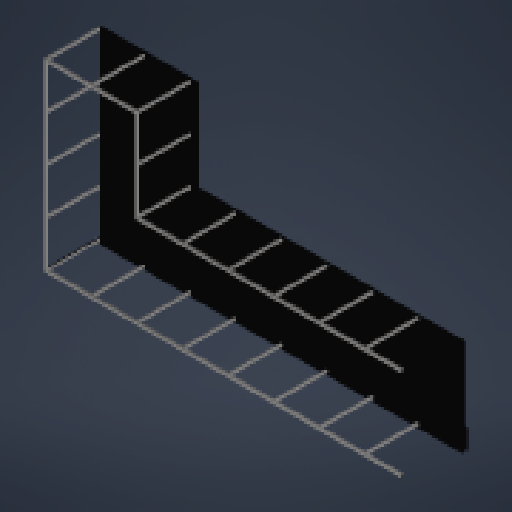
# Autodesk Inventor part: FirstFloorP
Saved by Autodesk Inventor 2025 (Build 290162000, 162)
## iProperties
Created: 2024-05-05
Part Number: FirstFloorP
Material: Generic
Document SubType Name: Modeling
Designer: zulet
Density: 1 g/cm^3
Appearance: Black
Author: zulet
Autodesk Inventor part; units mm, degrees
ref_plane "YZ Plane" through (0, 0, 0) normal (1, 0, 0) x (0, 1, 0)
ref_plane "XZ Plane" through (0, 0, 0) normal (0, 1, 0) x (-1, 0, 0)
ref_plane "XY Plane" through (0, 0, 0) normal (0, 0, 1) x (1, 0, 0)
sketch "Sketch1" plane through (0, 0, 0) normal (0, 0, 1) x (1, 0, 0)
  line L0 (7383.4617, 1848.5139) -> (5993.4617, 1848.5139) projected
  line L1 (7383.4617, 3293.5139) -> (7383.4617, 1793.5139) projected
  line L2 (7383.4617, 653.5139) -> (7383.4617, 1793.5139) projected
  line L3 (7353.4617, 653.5139) -> (7523.4617, 653.5139) projected
  line L4 (7416.4617, 640.8139) -> (7353.4617, 640.8139) projected
  arc A0 (7434.4617, 622.8139) -> (7416.4617, 640.8139) centre (7416.4617, 622.8139) ccw projected
  line L5 (7353.4617, 640.8139) -> (7353.4617, 653.5139) projected
  line L6 (7434.4617, 324.2139) -> (7434.4617, 622.8139) projected
  arc A1 (7416.4617, 306.2139) -> (7434.4617, 324.2139) centre (7416.4617, 324.2139) ccw projected
  line L7 (7416.4617, 306.2139) -> (7353.4617, 306.2139) projected
  line L8 (5938.4617, 348.5139) -> (7353.4617, 348.5139) construction
  line L9 (7353.4617, 238.5139) -> (7353.4617, 348.5139) projected
  line L10 (5938.4617, 238.5139) -> (7353.4617, 238.5139) projected
  line L11 (4438.4617, 238.5139) -> (5938.4617, 238.5139) projected
  line L12 (4438.4617, 238.5139) -> (2938.4617, 238.5139) projected
  line L13 (1438.4617, 238.5139) -> (2938.4617, 238.5139) projected
  line L14 (1383.4617, 1738.5139) -> (1383.4617, 348.5139) projected
  line L15 (1438.4617, 238.5139) -> (1438.4617, 348.5139) projected
  line L16 (1383.4617, 348.5139) -> (1493.4617, 348.5139) projected
  line L17 (1383.4617, 3238.5139) -> (1383.4617, 1848.5139) projected
  line L18 (2993.4617, 3348.5139) -> (1493.4617, 3348.5139) projected
  line L19 (2993.4617, 3238.5139) -> (2993.4617, 1848.5139) projected
  line L20 (2993.4617, 1848.5139) -> (4383.4617, 1848.5139) projected
  line L21 (4493.4617, 1848.5139) -> (5883.4617, 1848.5139) projected
  line L22 (1493.4617, 3348.5139) -> (1383.4617, 3348.5139)
  line L23 (1383.4617, 3348.5139) -> (1383.4617, 3238.5139)
  line L24 (1383.4617, 348.5139) -> (1383.4617, 238.5139)
  line L25 (1383.4617, 238.5139) -> (1438.4617, 238.5139)
  line L26 (2993.4617, 3348.5139) -> (2993.4617, 3238.5139)
  line L27 (4383.4617, 1848.5139) -> (4493.4617, 1848.5139)
  line L28 (5883.4617, 1848.5139) -> (5993.4617, 1848.5139)
  line L29 (1383.4617, 1848.5139) -> (1383.4617, 1738.5139)
  point P0 (0, 0)
  point P1 (7383.042, 1848.5139)
  point P2 (1472.0731, 342.554)
  constraints: 16 end point, 4 perpendicular, 1 collinear, 1 horizontal, 1 point on line, 1 vertical
extrude "Extrusion1" add sketch "Sketch1" along normal blind 20
sketch "Sketch2" plane through (0, 0, 20) normal (0, 0, 1) x (1, 0, 0)
  arc A0 (1423.4617, 286.5139) -> (1431.4617, 278.5139) centre (1431.4617, 286.5139) ccw projected
  line L0 (1423.4617, 286.5139) -> (1423.4617, 310.5139) projected
  arc A1 (1431.4617, 318.5139) -> (1423.4617, 310.5139) centre (1431.4617, 310.5139) ccw projected
  line L1 (1431.4617, 318.5139) -> (1455.4617, 318.5139) projected
  arc A2 (1463.4617, 310.5139) -> (1455.4617, 318.5139) centre (1455.4617, 310.5139) ccw projected
  line L2 (1463.4617, 310.5139) -> (1463.4617, 286.5139) projected
  arc A3 (1455.4617, 278.5139) -> (1463.4617, 286.5139) centre (1455.4617, 286.5139) ccw projected
  line L3 (1455.4617, 278.5139) -> (1431.4617, 278.5139) projected
  line L4 (1431.4617, 318.5139) -> (1455.4617, 318.5139)
  line L5 (1463.4617, 310.5139) -> (1463.4617, 286.5139)
  line L6 (1455.4617, 278.5139) -> (1431.4617, 278.5139)
  line L7 (1423.4617, 286.5139) -> (1423.4617, 310.5139)
  arc A4 (1431.4617, 318.5139) -> (1423.4617, 310.5139) centre (1431.4617, 310.5139) ccw
  arc A5 (1463.4617, 310.5139) -> (1455.4617, 318.5139) centre (1455.4617, 310.5139) ccw
  arc A6 (1455.4617, 278.5139) -> (1463.4617, 286.5139) centre (1455.4617, 286.5139) ccw
  arc A7 (1423.4617, 286.5139) -> (1431.4617, 278.5139) centre (1431.4617, 286.5139) ccw
  arc A8 (2205.4617, 278.5139) -> (2213.4617, 286.5139) centre (2205.4617, 286.5139) ccw
  line L8 (2205.4617, 278.5139) -> (2181.4617, 278.5139)
  line L9 (2213.4617, 310.5139) -> (2213.4617, 286.5139)
  arc A9 (2213.4617, 310.5139) -> (2205.4617, 318.5139) centre (2205.4617, 310.5139) ccw
  line L10 (2173.4617, 286.5139) -> (2173.4617, 310.5139)
  line L11 (2181.4617, 318.5139) -> (2205.4617, 318.5139)
  arc A10 (2181.4617, 318.5139) -> (2173.4617, 310.5139) centre (2181.4617, 310.5139) ccw
  arc A11 (2173.4617, 286.5139) -> (2181.4617, 278.5139) centre (2181.4617, 286.5139) ccw
  arc A12 (2955.4617, 278.5139) -> (2963.4617, 286.5139) centre (2955.4617, 286.5139) ccw
  line L12 (2955.4617, 278.5139) -> (2931.4617, 278.5139)
  line L13 (2963.4617, 310.5139) -> (2963.4617, 286.5139)
  arc A13 (2963.4617, 310.5139) -> (2955.4617, 318.5139) centre (2955.4617, 310.5139) ccw
  line L14 (2923.4617, 286.5139) -> (2923.4617, 310.5139)
  line L15 (2931.4617, 318.5139) -> (2955.4617, 318.5139)
  arc A14 (2931.4617, 318.5139) -> (2923.4617, 310.5139) centre (2931.4617, 310.5139) ccw
  arc A15 (2923.4617, 286.5139) -> (2931.4617, 278.5139) centre (2931.4617, 286.5139) ccw
  arc A16 (3705.4617, 278.5139) -> (3713.4617, 286.5139) centre (3705.4617, 286.5139) ccw
  line L16 (3705.4617, 278.5139) -> (3681.4617, 278.5139)
  line L17 (3713.4617, 310.5139) -> (3713.4617, 286.5139)
  arc A17 (3713.4617, 310.5139) -> (3705.4617, 318.5139) centre (3705.4617, 310.5139) ccw
  line L18 (3673.4617, 286.5139) -> (3673.4617, 310.5139)
  line L19 (3681.4617, 318.5139) -> (3705.4617, 318.5139)
  arc A18 (3681.4617, 318.5139) -> (3673.4617, 310.5139) centre (3681.4617, 310.5139) ccw
  arc A19 (3673.4617, 286.5139) -> (3681.4617, 278.5139) centre (3681.4617, 286.5139) ccw
  arc A20 (4455.4617, 278.5139) -> (4463.4617, 286.5139) centre (4455.4617, 286.5139) ccw
  line L20 (4455.4617, 278.5139) -> (4431.4617, 278.5139)
  line L21 (4463.4617, 310.5139) -> (4463.4617, 286.5139)
  arc A21 (4463.4617, 310.5139) -> (4455.4617, 318.5139) centre (4455.4617, 310.5139) ccw
  line L22 (4423.4617, 286.5139) -> (4423.4617, 310.5139)
  line L23 (4431.4617, 318.5139) -> (4455.4617, 318.5139)
  arc A22 (4431.4617, 318.5139) -> (4423.4617, 310.5139) centre (4431.4617, 310.5139) ccw
  arc A23 (4423.4617, 286.5139) -> (4431.4617, 278.5139) centre (4431.4617, 286.5139) ccw
  arc A24 (5205.4617, 278.5139) -> (5213.4617, 286.5139) centre (5205.4617, 286.5139) ccw
  line L24 (5205.4617, 278.5139) -> (5181.4617, 278.5139)
  line L25 (5213.4617, 310.5139) -> (5213.4617, 286.5139)
  arc A25 (5213.4617, 310.5139) -> (5205.4617, 318.5139) centre (5205.4617, 310.5139) ccw
  line L26 (5173.4617, 286.5139) -> (5173.4617, 310.5139)
  line L27 (5181.4617, 318.5139) -> (5205.4617, 318.5139)
  arc A26 (5181.4617, 318.5139) -> (5173.4617, 310.5139) centre (5181.4617, 310.5139) ccw
  arc A27 (5173.4617, 286.5139) -> (5181.4617, 278.5139) centre (5181.4617, 286.5139) ccw
  arc A28 (5955.4617, 278.5139) -> (5963.4617, 286.5139) centre (5955.4617, 286.5139) ccw
  line L28 (5955.4617, 278.5139) -> (5931.4617, 278.5139)
  line L29 (5963.4617, 310.5139) -> (5963.4617, 286.5139)
  arc A29 (5963.4617, 310.5139) -> (5955.4617, 318.5139) centre (5955.4617, 310.5139) ccw
  line L30 (5923.4617, 286.5139) -> (5923.4617, 310.5139)
  line L31 (5931.4617, 318.5139) -> (5955.4617, 318.5139)
  arc A30 (5931.4617, 318.5139) -> (5923.4617, 310.5139) centre (5931.4617, 310.5139) ccw
  arc A31 (5923.4617, 286.5139) -> (5931.4617, 278.5139) centre (5931.4617, 286.5139) ccw
  arc A32 (6705.4617, 278.5139) -> (6713.4617, 286.5139) centre (6705.4617, 286.5139) ccw
  line L32 (6705.4617, 278.5139) -> (6681.4617, 278.5139)
  line L33 (6713.4617, 310.5139) -> (6713.4617, 286.5139)
  arc A33 (6713.4617, 310.5139) -> (6705.4617, 318.5139) centre (6705.4617, 310.5139) ccw
  line L34 (6673.4617, 286.5139) -> (6673.4617, 310.5139)
  line L35 (6681.4617, 318.5139) -> (6705.4617, 318.5139)
  arc A34 (6681.4617, 318.5139) -> (6673.4617, 310.5139) centre (6681.4617, 310.5139) ccw
  arc A35 (6673.4617, 286.5139) -> (6681.4617, 278.5139) centre (6681.4617, 286.5139) ccw
  arc A36 (1455.4617, 1028.5139) -> (1463.4617, 1036.5139) centre (1455.4617, 1036.5139) ccw
  line L36 (1455.4617, 1028.5139) -> (1431.4617, 1028.5139)
  line L37 (1463.4617, 1060.5139) -> (1463.4617, 1036.5139)
  arc A37 (1463.4617, 1060.5139) -> (1455.4617, 1068.5139) centre (1455.4617, 1060.5139) ccw
  line L38 (1423.4617, 1036.5139) -> (1423.4617, 1060.5139)
  line L39 (1431.4617, 1068.5139) -> (1455.4617, 1068.5139)
  arc A38 (1431.4617, 1068.5139) -> (1423.4617, 1060.5139) centre (1431.4617, 1060.5139) ccw
  arc A39 (1423.4617, 1036.5139) -> (1431.4617, 1028.5139) centre (1431.4617, 1036.5139) ccw
  arc A40 (2205.4617, 1028.5139) -> (2213.4617, 1036.5139) centre (2205.4617, 1036.5139) ccw
  line L40 (2205.4617, 1028.5139) -> (2181.4617, 1028.5139)
  line L41 (2213.4617, 1060.5139) -> (2213.4617, 1036.5139)
  arc A41 (2213.4617, 1060.5139) -> (2205.4617, 1068.5139) centre (2205.4617, 1060.5139) ccw
  line L42 (2173.4617, 1036.5139) -> (2173.4617, 1060.5139)
  line L43 (2181.4617, 1068.5139) -> (2205.4617, 1068.5139)
  arc A42 (2181.4617, 1068.5139) -> (2173.4617, 1060.5139) centre (2181.4617, 1060.5139) ccw
  arc A43 (2173.4617, 1036.5139) -> (2181.4617, 1028.5139) centre (2181.4617, 1036.5139) ccw
  arc A44 (2955.4617, 1028.5139) -> (2963.4617, 1036.5139) centre (2955.4617, 1036.5139) ccw
  line L44 (2955.4617, 1028.5139) -> (2931.4617, 1028.5139)
  line L45 (2963.4617, 1060.5139) -> (2963.4617, 1036.5139)
  arc A45 (2963.4617, 1060.5139) -> (2955.4617, 1068.5139) centre (2955.4617, 1060.5139) ccw
  line L46 (2923.4617, 1036.5139) -> (2923.4617, 1060.5139)
  line L47 (2931.4617, 1068.5139) -> (2955.4617, 1068.5139)
  arc A46 (2931.4617, 1068.5139) -> (2923.4617, 1060.5139) centre (2931.4617, 1060.5139) ccw
  arc A47 (2923.4617, 1036.5139) -> (2931.4617, 1028.5139) centre (2931.4617, 1036.5139) ccw
  arc A48 (3705.4617, 1028.5139) -> (3713.4617, 1036.5139) centre (3705.4617, 1036.5139) ccw
  line L48 (3705.4617, 1028.5139) -> (3681.4617, 1028.5139)
  line L49 (3713.4617, 1060.5139) -> (3713.4617, 1036.5139)
  arc A49 (3713.4617, 1060.5139) -> (3705.4617, 1068.5139) centre (3705.4617, 1060.5139) ccw
  line L50 (3673.4617, 1036.5139) -> (3673.4617, 1060.5139)
  line L51 (3681.4617, 1068.5139) -> (3705.4617, 1068.5139)
  arc A50 (3681.4617, 1068.5139) -> (3673.4617, 1060.5139) centre (3681.4617, 1060.5139) ccw
  arc A51 (3673.4617, 1036.5139) -> (3681.4617, 1028.5139) centre (3681.4617, 1036.5139) ccw
  arc A52 (4455.4617, 1028.5139) -> (4463.4617, 1036.5139) centre (4455.4617, 1036.5139) ccw
  line L52 (4455.4617, 1028.5139) -> (4431.4617, 1028.5139)
  line L53 (4463.4617, 1060.5139) -> (4463.4617, 1036.5139)
  arc A53 (4463.4617, 1060.5139) -> (4455.4617, 1068.5139) centre (4455.4617, 1060.5139) ccw
  line L54 (4423.4617, 1036.5139) -> (4423.4617, 1060.5139)
  line L55 (4431.4617, 1068.5139) -> (4455.4617, 1068.5139)
  arc A54 (4431.4617, 1068.5139) -> (4423.4617, 1060.5139) centre (4431.4617, 1060.5139) ccw
  arc A55 (4423.4617, 1036.5139) -> (4431.4617, 1028.5139) centre (4431.4617, 1036.5139) ccw
  arc A56 (5205.4617, 1028.5139) -> (5213.4617, 1036.5139) centre (5205.4617, 1036.5139) ccw
  line L56 (5205.4617, 1028.5139) -> (5181.4617, 1028.5139)
  line L57 (5213.4617, 1060.5139) -> (5213.4617, 1036.5139)
  arc A57 (5213.4617, 1060.5139) -> (5205.4617, 1068.5139) centre (5205.4617, 1060.5139) ccw
  line L58 (5173.4617, 1036.5139) -> (5173.4617, 1060.5139)
  line L59 (5181.4617, 1068.5139) -> (5205.4617, 1068.5139)
  arc A58 (5181.4617, 1068.5139) -> (5173.4617, 1060.5139) centre (5181.4617, 1060.5139) ccw
  arc A59 (5173.4617, 1036.5139) -> (5181.4617, 1028.5139) centre (5181.4617, 1036.5139) ccw
  arc A60 (5955.4617, 1028.5139) -> (5963.4617, 1036.5139) centre (5955.4617, 1036.5139) ccw
  line L60 (5955.4617, 1028.5139) -> (5931.4617, 1028.5139)
  line L61 (5963.4617, 1060.5139) -> (5963.4617, 1036.5139)
  arc A61 (5963.4617, 1060.5139) -> (5955.4617, 1068.5139) centre (5955.4617, 1060.5139) ccw
  line L62 (5923.4617, 1036.5139) -> (5923.4617, 1060.5139)
  line L63 (5931.4617, 1068.5139) -> (5955.4617, 1068.5139)
  arc A62 (5931.4617, 1068.5139) -> (5923.4617, 1060.5139) centre (5931.4617, 1060.5139) ccw
  arc A63 (5923.4617, 1036.5139) -> (5931.4617, 1028.5139) centre (5931.4617, 1036.5139) ccw
  arc A64 (6705.4617, 1028.5139) -> (6713.4617, 1036.5139) centre (6705.4617, 1036.5139) ccw
  line L64 (6705.4617, 1028.5139) -> (6681.4617, 1028.5139)
  line L65 (6713.4617, 1060.5139) -> (6713.4617, 1036.5139)
  arc A65 (6713.4617, 1060.5139) -> (6705.4617, 1068.5139) centre (6705.4617, 1060.5139) ccw
  line L66 (6673.4617, 1036.5139) -> (6673.4617, 1060.5139)
  line L67 (6681.4617, 1068.5139) -> (6705.4617, 1068.5139)
  arc A66 (6681.4617, 1068.5139) -> (6673.4617, 1060.5139) centre (6681.4617, 1060.5139) ccw
  arc A67 (6673.4617, 1036.5139) -> (6681.4617, 1028.5139) centre (6681.4617, 1036.5139) ccw
  arc A68 (1455.4617, 1778.5139) -> (1463.4617, 1786.5139) centre (1455.4617, 1786.5139) ccw
  line L68 (1455.4617, 1778.5139) -> (1431.4617, 1778.5139)
  line L69 (1463.4617, 1810.5139) -> (1463.4617, 1786.5139)
  arc A69 (1463.4617, 1810.5139) -> (1455.4617, 1818.5139) centre (1455.4617, 1810.5139) ccw
  line L70 (1423.4617, 1786.5139) -> (1423.4617, 1810.5139)
  line L71 (1431.4617, 1818.5139) -> (1455.4617, 1818.5139)
  arc A70 (1431.4617, 1818.5139) -> (1423.4617, 1810.5139) centre (1431.4617, 1810.5139) ccw
  arc A71 (1423.4617, 1786.5139) -> (1431.4617, 1778.5139) centre (1431.4617, 1786.5139) ccw
  arc A72 (2205.4617, 1778.5139) -> (2213.4617, 1786.5139) centre (2205.4617, 1786.5139) ccw
  line L72 (2205.4617, 1778.5139) -> (2181.4617, 1778.5139)
  line L73 (2213.4617, 1810.5139) -> (2213.4617, 1786.5139)
  arc A73 (2213.4617, 1810.5139) -> (2205.4617, 1818.5139) centre (2205.4617, 1810.5139) ccw
  line L74 (2173.4617, 1786.5139) -> (2173.4617, 1810.5139)
  line L75 (2181.4617, 1818.5139) -> (2205.4617, 1818.5139)
  arc A74 (2181.4617, 1818.5139) -> (2173.4617, 1810.5139) centre (2181.4617, 1810.5139) ccw
  arc A75 (2173.4617, 1786.5139) -> (2181.4617, 1778.5139) centre (2181.4617, 1786.5139) ccw
  arc A76 (2955.4617, 1778.5139) -> (2963.4617, 1786.5139) centre (2955.4617, 1786.5139) ccw
  line L76 (2955.4617, 1778.5139) -> (2931.4617, 1778.5139)
  line L77 (2963.4617, 1810.5139) -> (2963.4617, 1786.5139)
  arc A77 (2963.4617, 1810.5139) -> (2955.4617, 1818.5139) centre (2955.4617, 1810.5139) ccw
  line L78 (2923.4617, 1786.5139) -> (2923.4617, 1810.5139)
  line L79 (2931.4617, 1818.5139) -> (2955.4617, 1818.5139)
  arc A78 (2931.4617, 1818.5139) -> (2923.4617, 1810.5139) centre (2931.4617, 1810.5139) ccw
  arc A79 (2923.4617, 1786.5139) -> (2931.4617, 1778.5139) centre (2931.4617, 1786.5139) ccw
  arc A80 (3705.4617, 1778.5139) -> (3713.4617, 1786.5139) centre (3705.4617, 1786.5139) ccw
  line L80 (3705.4617, 1778.5139) -> (3681.4617, 1778.5139)
  line L81 (3713.4617, 1810.5139) -> (3713.4617, 1786.5139)
  arc A81 (3713.4617, 1810.5139) -> (3705.4617, 1818.5139) centre (3705.4617, 1810.5139) ccw
  line L82 (3673.4617, 1786.5139) -> (3673.4617, 1810.5139)
  line L83 (3681.4617, 1818.5139) -> (3705.4617, 1818.5139)
  arc A82 (3681.4617, 1818.5139) -> (3673.4617, 1810.5139) centre (3681.4617, 1810.5139) ccw
  arc A83 (3673.4617, 1786.5139) -> (3681.4617, 1778.5139) centre (3681.4617, 1786.5139) ccw
  arc A84 (4455.4617, 1778.5139) -> (4463.4617, 1786.5139) centre (4455.4617, 1786.5139) ccw
  line L84 (4455.4617, 1778.5139) -> (4431.4617, 1778.5139)
  line L85 (4463.4617, 1810.5139) -> (4463.4617, 1786.5139)
  arc A85 (4463.4617, 1810.5139) -> (4455.4617, 1818.5139) centre (4455.4617, 1810.5139) ccw
  line L86 (4423.4617, 1786.5139) -> (4423.4617, 1810.5139)
  line L87 (4431.4617, 1818.5139) -> (4455.4617, 1818.5139)
  arc A86 (4431.4617, 1818.5139) -> (4423.4617, 1810.5139) centre (4431.4617, 1810.5139) ccw
  arc A87 (4423.4617, 1786.5139) -> (4431.4617, 1778.5139) centre (4431.4617, 1786.5139) ccw
  arc A88 (5205.4617, 1778.5139) -> (5213.4617, 1786.5139) centre (5205.4617, 1786.5139) ccw
  line L88 (5205.4617, 1778.5139) -> (5181.4617, 1778.5139)
  line L89 (5213.4617, 1810.5139) -> (5213.4617, 1786.5139)
  arc A89 (5213.4617, 1810.5139) -> (5205.4617, 1818.5139) centre (5205.4617, 1810.5139) ccw
  line L90 (5173.4617, 1786.5139) -> (5173.4617, 1810.5139)
  line L91 (5181.4617, 1818.5139) -> (5205.4617, 1818.5139)
  arc A90 (5181.4617, 1818.5139) -> (5173.4617, 1810.5139) centre (5181.4617, 1810.5139) ccw
  arc A91 (5173.4617, 1786.5139) -> (5181.4617, 1778.5139) centre (5181.4617, 1786.5139) ccw
  arc A92 (5955.4617, 1778.5139) -> (5963.4617, 1786.5139) centre (5955.4617, 1786.5139) ccw
  line L92 (5955.4617, 1778.5139) -> (5931.4617, 1778.5139)
  line L93 (5963.4617, 1810.5139) -> (5963.4617, 1786.5139)
  arc A93 (5963.4617, 1810.5139) -> (5955.4617, 1818.5139) centre (5955.4617, 1810.5139) ccw
  line L94 (5923.4617, 1786.5139) -> (5923.4617, 1810.5139)
  line L95 (5931.4617, 1818.5139) -> (5955.4617, 1818.5139)
  arc A94 (5931.4617, 1818.5139) -> (5923.4617, 1810.5139) centre (5931.4617, 1810.5139) ccw
  arc A95 (5923.4617, 1786.5139) -> (5931.4617, 1778.5139) centre (5931.4617, 1786.5139) ccw
  arc A96 (6705.4617, 1778.5139) -> (6713.4617, 1786.5139) centre (6705.4617, 1786.5139) ccw
  line L96 (6705.4617, 1778.5139) -> (6681.4617, 1778.5139)
  line L97 (6713.4617, 1810.5139) -> (6713.4617, 1786.5139)
  arc A97 (6713.4617, 1810.5139) -> (6705.4617, 1818.5139) centre (6705.4617, 1810.5139) ccw
  line L98 (6673.4617, 1786.5139) -> (6673.4617, 1810.5139)
  line L99 (6681.4617, 1818.5139) -> (6705.4617, 1818.5139)
  arc A98 (6681.4617, 1818.5139) -> (6673.4617, 1810.5139) centre (6681.4617, 1810.5139) ccw
  arc A99 (6673.4617, 1786.5139) -> (6681.4617, 1778.5139) centre (6681.4617, 1786.5139) ccw
  arc A100 (1455.4617, 2528.5139) -> (1463.4617, 2536.5139) centre (1455.4617, 2536.5139) ccw
  line L100 (1455.4617, 2528.5139) -> (1431.4617, 2528.5139)
  line L101 (1463.4617, 2560.5139) -> (1463.4617, 2536.5139)
  arc A101 (1463.4617, 2560.5139) -> (1455.4617, 2568.5139) centre (1455.4617, 2560.5139) ccw
  line L102 (1423.4617, 2536.5139) -> (1423.4617, 2560.5139)
  line L103 (1431.4617, 2568.5139) -> (1455.4617, 2568.5139)
  arc A102 (1431.4617, 2568.5139) -> (1423.4617, 2560.5139) centre (1431.4617, 2560.5139) ccw
  arc A103 (1423.4617, 2536.5139) -> (1431.4617, 2528.5139) centre (1431.4617, 2536.5139) ccw
  arc A104 (2205.4617, 2528.5139) -> (2213.4617, 2536.5139) centre (2205.4617, 2536.5139) ccw
  line L104 (2205.4617, 2528.5139) -> (2181.4617, 2528.5139)
  line L105 (2213.4617, 2560.5139) -> (2213.4617, 2536.5139)
  arc A105 (2213.4617, 2560.5139) -> (2205.4617, 2568.5139) centre (2205.4617, 2560.5139) ccw
  line L106 (2173.4617, 2536.5139) -> (2173.4617, 2560.5139)
  line L107 (2181.4617, 2568.5139) -> (2205.4617, 2568.5139)
  arc A106 (2181.4617, 2568.5139) -> (2173.4617, 2560.5139) centre (2181.4617, 2560.5139) ccw
  arc A107 (2173.4617, 2536.5139) -> (2181.4617, 2528.5139) centre (2181.4617, 2536.5139) ccw
  arc A108 (2955.4617, 2528.5139) -> (2963.4617, 2536.5139) centre (2955.4617, 2536.5139) ccw
  line L108 (2955.4617, 2528.5139) -> (2931.4617, 2528.5139)
  line L109 (2963.4617, 2560.5139) -> (2963.4617, 2536.5139)
  arc A109 (2963.4617, 2560.5139) -> (2955.4617, 2568.5139) centre (2955.4617, 2560.5139) ccw
  line L110 (2923.4617, 2536.5139) -> (2923.4617, 2560.5139)
  line L111 (2931.4617, 2568.5139) -> (2955.4617, 2568.5139)
  arc A110 (2931.4617, 2568.5139) -> (2923.4617, 2560.5139) centre (2931.4617, 2560.5139) ccw
  arc A111 (2923.4617, 2536.5139) -> (2931.4617, 2528.5139) centre (2931.4617, 2536.5139) ccw
  arc A112 (3705.4617, 2528.5139) -> (3713.4617, 2536.5139) centre (3705.4617, 2536.5139) ccw
  line L112 (3705.4617, 2528.5139) -> (3681.4617, 2528.5139)
  line L113 (3713.4617, 2560.5139) -> (3713.4617, 2536.5139)
  arc A113 (3713.4617, 2560.5139) -> (3705.4617, 2568.5139) centre (3705.4617, 2560.5139) ccw
  line L114 (3673.4617, 2536.5139) -> (3673.4617, 2560.5139)
  line L115 (3681.4617, 2568.5139) -> (3705.4617, 2568.5139)
  arc A114 (3681.4617, 2568.5139) -> (3673.4617, 2560.5139) centre (3681.4617, 2560.5139) ccw
  arc A115 (3673.4617, 2536.5139) -> (3681.4617, 2528.5139) centre (3681.4617, 2536.5139) ccw
  arc A116 (4455.4617, 2528.5139) -> (4463.4617, 2536.5139) centre (4455.4617, 2536.5139) ccw
  line L116 (4455.4617, 2528.5139) -> (4431.4617, 2528.5139)
  line L117 (4463.4617, 2560.5139) -> (4463.4617, 2536.5139)
  arc A117 (4463.4617, 2560.5139) -> (4455.4617, 2568.5139) centre (4455.4617, 2560.5139) ccw
  line L118 (4423.4617, 2536.5139) -> (4423.4617, 2560.5139)
  line L119 (4431.4617, 2568.5139) -> (4455.4617, 2568.5139)
  arc A118 (4431.4617, 2568.5139) -> (4423.4617, 2560.5139) centre (4431.4617, 2560.5139) ccw
  arc A119 (4423.4617, 2536.5139) -> (4431.4617, 2528.5139) centre (4431.4617, 2536.5139) ccw
  arc A120 (5205.4617, 2528.5139) -> (5213.4617, 2536.5139) centre (5205.4617, 2536.5139) ccw
  line L120 (5205.4617, 2528.5139) -> (5181.4617, 2528.5139)
  line L121 (5213.4617, 2560.5139) -> (5213.4617, 2536.5139)
  arc A121 (5213.4617, 2560.5139) -> (5205.4617, 2568.5139) centre (5205.4617, 2560.5139) ccw
  line L122 (5173.4617, 2536.5139) -> (5173.4617, 2560.5139)
  line L123 (5181.4617, 2568.5139) -> (5205.4617, 2568.5139)
  arc A122 (5181.4617, 2568.5139) -> (5173.4617, 2560.5139) centre (5181.4617, 2560.5139) ccw
  arc A123 (5173.4617, 2536.5139) -> (5181.4617, 2528.5139) centre (5181.4617, 2536.5139) ccw
  arc A124 (5955.4617, 2528.5139) -> (5963.4617, 2536.5139) centre (5955.4617, 2536.5139) ccw
  line L124 (5955.4617, 2528.5139) -> (5931.4617, 2528.5139)
  line L125 (5963.4617, 2560.5139) -> (5963.4617, 2536.5139)
  arc A125 (5963.4617, 2560.5139) -> (5955.4617, 2568.5139) centre (5955.4617, 2560.5139) ccw
  line L126 (5923.4617, 2536.5139) -> (5923.4617, 2560.5139)
  line L127 (5931.4617, 2568.5139) -> (5955.4617, 2568.5139)
  arc A126 (5931.4617, 2568.5139) -> (5923.4617, 2560.5139) centre (5931.4617, 2560.5139) ccw
  arc A127 (5923.4617, 2536.5139) -> (5931.4617, 2528.5139) centre (5931.4617, 2536.5139) ccw
  arc A128 (6705.4617, 2528.5139) -> (6713.4617, 2536.5139) centre (6705.4617, 2536.5139) ccw
  line L128 (6705.4617, 2528.5139) -> (6681.4617, 2528.5139)
  line L129 (6713.4617, 2560.5139) -> (6713.4617, 2536.5139)
  arc A129 (6713.4617, 2560.5139) -> (6705.4617, 2568.5139) centre (6705.4617, 2560.5139) ccw
  line L130 (6673.4617, 2536.5139) -> (6673.4617, 2560.5139)
  line L131 (6681.4617, 2568.5139) -> (6705.4617, 2568.5139)
  arc A130 (6681.4617, 2568.5139) -> (6673.4617, 2560.5139) centre (6681.4617, 2560.5139) ccw
  arc A131 (6673.4617, 2536.5139) -> (6681.4617, 2528.5139) centre (6681.4617, 2536.5139) ccw
  arc A132 (1455.4617, 3278.5139) -> (1463.4617, 3286.5139) centre (1455.4617, 3286.5139) ccw
  line L132 (1455.4617, 3278.5139) -> (1431.4617, 3278.5139)
  line L133 (1463.4617, 3310.5139) -> (1463.4617, 3286.5139)
  arc A133 (1463.4617, 3310.5139) -> (1455.4617, 3318.5139) centre (1455.4617, 3310.5139) ccw
  line L134 (1423.4617, 3286.5139) -> (1423.4617, 3310.5139)
  line L135 (1431.4617, 3318.5139) -> (1455.4617, 3318.5139)
  arc A134 (1431.4617, 3318.5139) -> (1423.4617, 3310.5139) centre (1431.4617, 3310.5139) ccw
  arc A135 (1423.4617, 3286.5139) -> (1431.4617, 3278.5139) centre (1431.4617, 3286.5139) ccw
  arc A136 (2205.4617, 3278.5139) -> (2213.4617, 3286.5139) centre (2205.4617, 3286.5139) ccw
  line L136 (2205.4617, 3278.5139) -> (2181.4617, 3278.5139)
  line L137 (2213.4617, 3310.5139) -> (2213.4617, 3286.5139)
  arc A137 (2213.4617, 3310.5139) -> (2205.4617, 3318.5139) centre (2205.4617, 3310.5139) ccw
  line L138 (2173.4617, 3286.5139) -> (2173.4617, 3310.5139)
  line L139 (2181.4617, 3318.5139) -> (2205.4617, 3318.5139)
  arc A138 (2181.4617, 3318.5139) -> (2173.4617, 3310.5139) centre (2181.4617, 3310.5139) ccw
  arc A139 (2173.4617, 3286.5139) -> (2181.4617, 3278.5139) centre (2181.4617, 3286.5139) ccw
  arc A140 (2955.4617, 3278.5139) -> (2963.4617, 3286.5139) centre (2955.4617, 3286.5139) ccw
  line L140 (2955.4617, 3278.5139) -> (2931.4617, 3278.5139)
  line L141 (2963.4617, 3310.5139) -> (2963.4617, 3286.5139)
  arc A141 (2963.4617, 3310.5139) -> (2955.4617, 3318.5139) centre (2955.4617, 3310.5139) ccw
  line L142 (2923.4617, 3286.5139) -> (2923.4617, 3310.5139)
  line L143 (2931.4617, 3318.5139) -> (2955.4617, 3318.5139)
  arc A142 (2931.4617, 3318.5139) -> (2923.4617, 3310.5139) centre (2931.4617, 3310.5139) ccw
  arc A143 (2923.4617, 3286.5139) -> (2931.4617, 3278.5139) centre (2931.4617, 3286.5139) ccw
  arc A144 (3705.4617, 3278.5139) -> (3713.4617, 3286.5139) centre (3705.4617, 3286.5139) ccw
  line L144 (3705.4617, 3278.5139) -> (3681.4617, 3278.5139)
  line L145 (3713.4617, 3310.5139) -> (3713.4617, 3286.5139)
  arc A145 (3713.4617, 3310.5139) -> (3705.4617, 3318.5139) centre (3705.4617, 3310.5139) ccw
  line L146 (3673.4617, 3286.5139) -> (3673.4617, 3310.5139)
  line L147 (3681.4617, 3318.5139) -> (3705.4617, 3318.5139)
  arc A146 (3681.4617, 3318.5139) -> (3673.4617, 3310.5139) centre (3681.4617, 3310.5139) ccw
  arc A147 (3673.4617, 3286.5139) -> (3681.4617, 3278.5139) centre (3681.4617, 3286.5139) ccw
  arc A148 (4455.4617, 3278.5139) -> (4463.4617, 3286.5139) centre (4455.4617, 3286.5139) ccw
  line L148 (4455.4617, 3278.5139) -> (4431.4617, 3278.5139)
  line L149 (4463.4617, 3310.5139) -> (4463.4617, 3286.5139)
  arc A149 (4463.4617, 3310.5139) -> (4455.4617, 3318.5139) centre (4455.4617, 3310.5139) ccw
  line L150 (4423.4617, 3286.5139) -> (4423.4617, 3310.5139)
  line L151 (4431.4617, 3318.5139) -> (4455.4617, 3318.5139)
  arc A150 (4431.4617, 3318.5139) -> (4423.4617, 3310.5139) centre (4431.4617, 3310.5139) ccw
  arc A151 (4423.4617, 3286.5139) -> (4431.4617, 3278.5139) centre (4431.4617, 3286.5139) ccw
  arc A152 (5205.4617, 3278.5139) -> (5213.4617, 3286.5139) centre (5205.4617, 3286.5139) ccw
  line L152 (5205.4617, 3278.5139) -> (5181.4617, 3278.5139)
  line L153 (5213.4617, 3310.5139) -> (5213.4617, 3286.5139)
  arc A153 (5213.4617, 3310.5139) -> (5205.4617, 3318.5139) centre (5205.4617, 3310.5139) ccw
  line L154 (5173.4617, 3286.5139) -> (5173.4617, 3310.5139)
  line L155 (5181.4617, 3318.5139) -> (5205.4617, 3318.5139)
  arc A154 (5181.4617, 3318.5139) -> (5173.4617, 3310.5139) centre (5181.4617, 3310.5139) ccw
  arc A155 (5173.4617, 3286.5139) -> (5181.4617, 3278.5139) centre (5181.4617, 3286.5139) ccw
  arc A156 (5955.4617, 3278.5139) -> (5963.4617, 3286.5139) centre (5955.4617, 3286.5139) ccw
  line L156 (5955.4617, 3278.5139) -> (5931.4617, 3278.5139)
  line L157 (5963.4617, 3310.5139) -> (5963.4617, 3286.5139)
  arc A157 (5963.4617, 3310.5139) -> (5955.4617, 3318.5139) centre (5955.4617, 3310.5139) ccw
  line L158 (5923.4617, 3286.5139) -> (5923.4617, 3310.5139)
  line L159 (5931.4617, 3318.5139) -> (5955.4617, 3318.5139)
  arc A158 (5931.4617, 3318.5139) -> (5923.4617, 3310.5139) centre (5931.4617, 3310.5139) ccw
  arc A159 (5923.4617, 3286.5139) -> (5931.4617, 3278.5139) centre (5931.4617, 3286.5139) ccw
  arc A160 (6705.4617, 3278.5139) -> (6713.4617, 3286.5139) centre (6705.4617, 3286.5139) ccw
  line L160 (6705.4617, 3278.5139) -> (6681.4617, 3278.5139)
  line L161 (6713.4617, 3310.5139) -> (6713.4617, 3286.5139)
  arc A161 (6713.4617, 3310.5139) -> (6705.4617, 3318.5139) centre (6705.4617, 3310.5139) ccw
  line L162 (6673.4617, 3286.5139) -> (6673.4617, 3310.5139)
  line L163 (6681.4617, 3318.5139) -> (6705.4617, 3318.5139)
  arc A162 (6681.4617, 3318.5139) -> (6673.4617, 3310.5139) centre (6681.4617, 3310.5139) ccw
  arc A163 (6673.4617, 3286.5139) -> (6681.4617, 3278.5139) centre (6681.4617, 3286.5139) ccw
  point P0 (0, 0)
  point P1 (1423.4617, 318.5139)
  point P2 (2173.4617, 318.5139)
  point P3 (2923.4617, 318.5139)
  point P4 (3673.4617, 318.5139)
  point P5 (4423.4617, 318.5139)
  point P6 (5173.4617, 318.5139)
  point P7 (5923.4617, 318.5139)
  point P8 (6673.4617, 318.5139)
  point P9 (1423.4617, 1068.5139)
  point P10 (2173.4617, 1068.5139)
  point P11 (2923.4617, 1068.5139)
  point P12 (3673.4617, 1068.5139)
  point P13 (4423.4617, 1068.5139)
  point P14 (5173.4617, 1068.5139)
  point P15 (5923.4617, 1068.5139)
  point P16 (6673.4617, 1068.5139)
  point P17 (1423.4617, 1818.5139)
  point P18 (2173.4617, 1818.5139)
  point P19 (2923.4617, 1818.5139)
  point P20 (3673.4617, 1818.5139)
  point P21 (4423.4617, 1818.5139)
  point P22 (5173.4617, 1818.5139)
  point P23 (5923.4617, 1818.5139)
  point P24 (6673.4617, 1818.5139)
  point P25 (1423.4617, 2568.5139)
  point P26 (2173.4617, 2568.5139)
  point P27 (2923.4617, 2568.5139)
  point P28 (3673.4617, 2568.5139)
  point P29 (4423.4617, 2568.5139)
  point P30 (5173.4617, 2568.5139)
  point P31 (5923.4617, 2568.5139)
  point P32 (6673.4617, 2568.5139)
  point P33 (1423.4617, 3318.5139)
  point P34 (2173.4617, 3318.5139)
  point P35 (2923.4617, 3318.5139)
  point P36 (3673.4617, 3318.5139)
  point P37 (4423.4617, 3318.5139)
  point P38 (5173.4617, 3318.5139)
  point P39 (5923.4617, 3318.5139)
  point P40 (6673.4617, 3318.5139)
  point P41 (1375.4617, 278.5139)
  point P42 (1455.4617, 278.5139)
  dimension "d2" = 8
  dimension "d5" = 750
  dimension "d8" = 750
  constraints: 320 end point, 320 point on circle, 160 centre point, 82 point on line, 8 tangent, 3 collinear, 3 equal radius, 2 horizontal, 2 parallel, 1 perpendicular, 1 vertical, 818 other
  measures "d2" radius of A4
  measures "d5" distance of A6.centre A8.centre
  measures "d8" distance of A6.centre A36.centre
extrude "Extrusion2" add sketch "Sketch2" along normal blind 850 contours L0 A1 L1 A2 L2 A3 L3 A0 | L8 A11 L10 A10 L11 A9 L9 A8 | L12 A15 L14 A14 L15 A13 L13 A12 | L16 A19 L18 A18 L19 A17 L17 A16 | L20 A23 L22 A22 L23 A21 L21 A20 | L24 A27 L26 A26 L27 A25 L25 A24 | L28 A31 L30 A30 L31 A29 L29 A28 | L32 A35 L34 A34 L35 A33 L33 A32 | L36 A39 L38 A38 L39 A37 L37 A36 | L68 A71 L70 A70 L71 A69 L69 A68 | L76 A79 L78 A78 L79 A77 L77 A76 | L80 A83 L82 A82 L83 A81 L81 A80 | L84 A87 L86 A86 L87 A85 L85 A84 | L88 A91 L90 A90 L91 A89 L89 A88 | L92 A95 L94 A94 L95 A93 L93 A92 | L96 A99 L98 A98 L99 A97 L97 A96 | L100 A103 L102 A102 L103 A101 L101 A100 | L108 A111 L110 A110 L111 A109 L109 A108 | L132 A135 L134 A134 L135 A133 L133 A132 | L136 A139 L138 A138 L139 A137 L137 A136 | L140 A143 L142 A142 L143 A141 L141 A140
sketch "Sketch3" plane through (0, 0, 870) normal (0, 0, 1) x (1, 0, 0)
  line L0 (1423.4617, 278.5139) -> (1463.4617, 278.5139)
  line L1 (1463.4617, 278.5139) -> (1463.4617, 3318.5139)
  line L2 (1463.4617, 3318.5139) -> (1423.4617, 3318.5139)
  line L3 (1423.4617, 3318.5139) -> (1423.4617, 278.5139)
  line L4 (1431.4617, 278.5139) -> (1423.4617, 278.5139) construction
  arc A0 (1423.4617, 286.5139) -> (1431.4617, 278.5139) centre (1431.4617, 286.5139) ccw construction
  line L5 (1423.4617, 278.5139) -> (1423.4617, 286.5139) construction
  line L6 (1423.4617, 278.5139) -> (7323.4617, 278.5139)
  line L7 (7323.4617, 278.5139) -> (7323.4617, 318.5139)
  line L8 (7323.4617, 318.5139) -> (1423.4617, 318.5139)
  line L9 (1423.4617, 318.5139) -> (1423.4617, 278.5139)
  line L10 (1423.4617, 3318.5139) -> (2963.4617, 3318.5139)
  line L11 (2963.4617, 3318.5139) -> (2963.4617, 3278.5139)
  line L12 (2963.4617, 3278.5139) -> (1423.4617, 3278.5139)
  line L13 (1423.4617, 3278.5139) -> (1423.4617, 3318.5139)
  line L14 (2963.4617, 3318.5139) -> (2923.4617, 3318.5139)
  line L15 (2923.4617, 3318.5139) -> (2923.4617, 1778.5139)
  line L16 (2923.4617, 1778.5139) -> (2963.4617, 1778.5139)
  line L17 (2963.4617, 1778.5139) -> (2963.4617, 3318.5139)
  line L18 (2923.4617, 1778.5139) -> (7323.4617, 1778.5139)
  line L19 (7323.4617, 1778.5139) -> (7323.4617, 1818.5139)
  line L20 (7323.4617, 1818.5139) -> (2923.4617, 1818.5139)
  line L21 (2923.4617, 1818.5139) -> (2923.4617, 1778.5139)
  arc A1 (1423.4617, 286.5139) -> (1431.4617, 278.5139) centre (1431.4617, 286.5139) ccw projected
  line L22 (1431.4617, 286.5139) -> (1431.4617, 278.5139) construction
  line L23 (1431.4617, 286.5139) -> (1423.4617, 286.5139) construction
  point P0 (0, 0)
  point P1 (2963.4617, 1818.5139)
  point P2 (1463.4617, 318.5139)
  point P3 (1463.4617, 3278.5139)
  point P4 (2923.4617, 3278.5139)
  dimension "d13" = 40
  dimension "d14" = 3040
  dimension "d15" = 5900
  dimension "d16" = 40
  dimension "d17" = 1540
  dimension "d18" = 40
  dimension "d19" = 40
  dimension "d20" = 1540
  dimension "d21" = 4400
  dimension "d22" = 40
  dimension "d25" = 8
  dimension "d26" = 8
  constraints: 48 end point, 10 parallel, 7 perpendicular, 6 horizontal, 2 point on circle, 1 centre point, 1 coincident, 1 point on line, 1 vertical
  measures "d13" distance of L2.end L1.end
  measures "d14" distance of L1.end L0.end
  measures "d15" distance of L8.end L7.end
  measures "d16" distance of L7.end L6.end
  measures "d17" distance of L11.end L12.end
  measures "d18" distance of L10.end L11.end
  measures "d19" distance of L16.end L15.end
  measures "d20" distance of L15.end L14.end
  measures "d21" distance of L20.end L19.end
  measures "d22" distance of L19.end L18.end
  measures "d25" radius of A0
  measures "d26" distance of L23.start L23.end
extrude "Extrusion3" add sketch "Sketch3" along normal blind 40
equation "\"d26\" = d25"
body "Solid1"
